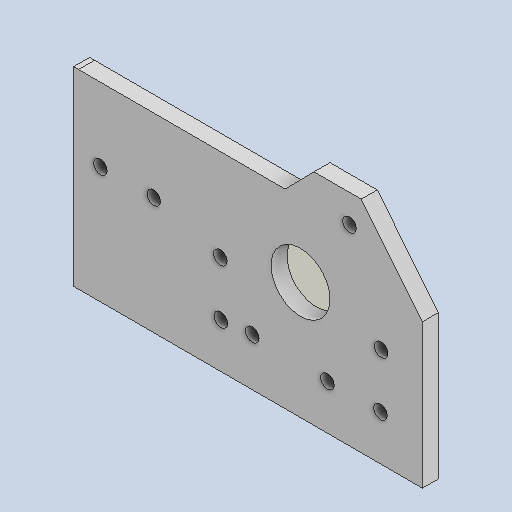
# Autodesk Inventor part: X axis motor mount
Saved by Autodesk Inventor 2023.2 (Build 272271000, 271)
## iProperties
Created: 2023-04-13
Part Number: X axis motor mount
Material: Generic
Document SubType Name: Modeling
Designer: dmargari
Density: 1 g/cm^3
Appearance: Default
Author: dmargari
## iProperties of the stored document X axis motor mount_3DPrint.ipt
Created: 2023-04-13
Part Number: X axis motor mount_3DPrint
Material: Generic
Document SubType Name: Modeling
Designer: dmargari
Density: 1 g/cm^3
Appearance: Default
Author: dmargari
Autodesk Inventor part; units mm, degrees
ref_plane "YZ Plane" through (0, 0, 0) normal (1, 0, 0) x (0, 1, 0)
ref_plane "XZ Plane" through (0, 0, 0) normal (0, 1, 0) x (-1, 0, 0)
ref_plane "XY Plane" through (0, 0, 0) normal (0, 0, 1) x (1, 0, 0)
ref_plane "Work Plane1" through (-0.0001, 0, -396.2798) normal (0.0000002, 0, 1) x (1, 0.0000006, -0.0000002)
sketch "Sketch1" plane through (-0.0001, 0, -396.2798) normal (0.0000002, 0, 1) x (1, 0.0000006, -0.0000002)
  circle A0 centre (29.9617, 10.0469) radius 2.1 projected
  circle A1 centre (29.9617, -9.9531) radius 2.1 projected
  circle A2 centre (-30.0383, -9.9531) radius 2.1 projected
  circle A3 centre (-30.0383, 10.0469) radius 2.1 projected
  circle A4 centre (-10.0383, -9.9531) radius 2.1 projected
  circle A5 centre (9.9617, -9.9531) radius 2.1 projected
  line L0 (39.9617, 19.5469) -> (39.9617, 14.8783) projected
  line L1 (39.9617, -14.7846) -> (39.9617, -19.4531) projected
  line L2 (39.4617, -19.9531) -> (34.7932, -19.9531) projected
  line L3 (20.4617, 20.0469) -> (25.0617, 20.0469) projected
  line L4 (-34.8697, -19.9531) -> (-39.5383, -19.9531) projected
  line L5 (-40.0383, 14.8783) -> (-40.0383, 19.5469) projected
  line L6 (-39.5383, 20.0469) -> (-34.9383, 20.0469) projected
  line L7 (-40.0383, -19.4531) -> (-40.0383, -14.7846) projected
  line L8 (39.9617, 20.0469) -> (39.9617, -19.9532) construction
  line L9 (39.9617, -19.9532) -> (-40.0383, -19.9531) construction
  line L10 (-40.0383, -19.9531) -> (-40.0383, 20.0469) construction
  line L11 (-20.0383, 19.5469) -> (-20.0383, 14.8783) projected
  line L12 (19.9617, 0.0469) -> (19.9617, 5.2154) projected
  line L13 (-20.0383, 0.0469) -> (-14.9383, 0.0469) projected
  line L14 (39.9617, 20.0469) -> (19.9617, 20.0469) construction
  line L15 (19.9617, 20.0469) -> (19.9617, 0.0469) construction
  line L16 (-20.0383, 0.0469) -> (19.9617, 0.0469) construction
  line L17 (-40.0383, 20.0469) -> (-20.0383, 20.0469) construction
  line L18 (-20.0383, 20.0469) -> (-20.0383, 0.0469) construction
  line L19 (45.6493, 27.0762) -> (45.6493, -26.9238)
  line L20 (-64.252, 0) -> (79.446, 0) construction
  line L21 (18.0586, 45.1257) -> (28.1307, -1.0304) construction
  line L22 (28.1307, -1.0304) -> (-18.0254, -11.1025) construction
  circle A6 centre (28.1307, -1.0304) radius 2.55
  circle A7 centre (-18.0452, -9.0596) radius 2.55
  circle A8 centre (18.0586, 45.1257) radius 2.55
  circle A9 centre (-18.0452, -9.0596) radius 3.5 construction
  circle A10 centre (18.0586, 45.1257) radius 3.5 construction
  circle A11 centre (28.1307, -1.0304) radius 3.5 construction
  line L23 (48.593, 17.0469) -> (-85.0986, 17.0469) construction
  line L24 (-0.0383, 40.3857) -> (-0.0383, -33.3677) construction
  circle A12 centre (-0.0383, 17.0469) radius 11.05
  line L25 (45.6493, 27.0762) -> (22.7125, 55.4148)
  line L26 (22.7125, 55.4148) -> (5.0035, 55.4148)
  line L27 (5.0035, 55.4148) -> (-5.8027, 44.4325)
  line L28 (-64.3507, 44.498) -> (-5.8027, 44.4325)
  line L29 (-64.3507, 44.498) -> (-66.5209, 44.5005)
  line L30 (-55.0383, 44.4876) -> (-55.0383, -55.6033) construction
  line L31 (45.6493, -26.9238) -> (-85.0986, -26.7776)
  line L32 (45.6493, -26.9238) -> (185.0342, -26.9238) construction
  line L33 (40.0498, -55.6502) -> (39.9617, -55.6502)
  line L34 (-83.2302, 44.5192) -> (-66.5209, 44.5005)
  line L35 (-85.0986, -26.7776) -> (-85.0986, 44.5192)
  line L36 (-85.0986, 44.5192) -> (-83.2302, 44.5192)
  point P0 (0, 0)
  point P1 (0, 17)
  point P2 (22.7617, 20.0469)
  point P3 (19.9617, 2.6311)
  point P4 (-40.0383, -17.1189)
  point P5 (-55.0383, -5.5579)
  point P6 (-75.0383, 17.0469)
  point P7 (-55.0383, 17.0469)
  dimension "d2" = 110
  dimension "d3" = 5.1
  dimension "d4" = 5.1
  dimension "d5" = 5.1
  dimension "d7" = 7
  dimension "d8" = 7
  dimension "d9" = 7
  dimension "d10" = 3
  dimension "d11" = 20
  dimension "d12" = 22.1
  dimension "d30" = 15
  dimension "d33" = 54
  dimension "d36" = 20
  dimension "d37" = 15
  constraints: 52 end point, 13 coincident, 13 point on line, 7 centre point, 7 perpendicular, 4 horizontal, 4 midpoint, 2 vertical, 1 collinear
  measures "d2" horizontal distance of L28.start L19.start
  measures "d3" diameter of A6
  measures "d4" diameter of A7
  measures "d5" diameter of A8
  measures "d7" diameter of A9
  measures "d8" diameter of A10
  measures "d9" diameter of A11
  measures "d10" distance from line of point (22.762, 20.047) L23
  measures "d11" distance from line of point (19.962, 2.631) L24
  measures "d12" diameter of A12
  measures "d30" distance from line of point (-40.038, -17.119) L30
  measures "d33" distance of L19.start L19.end
  measures "d36" distance of point (-55.038, 17.047) point (-75.038, 17.047)
  measures "d37" distance from line of L10 point (-55.038, 17.047)
extrude "Extrusion1" add sketch "Sketch1" along normal blind 6 contours A0 | A1 | A2 | A3 | A4 | A5 | L19 L31 L35 L36 L34 L29 L28 L27 L26 L25 | A6 | A7 | A8
sketch "Sketch2" plane through (-0.0001, 0, -396.2798) normal (-0.0000002, 0, -1) x (-1, -0.0000006, 0.0000002)
  point P0 (0, 0)
  point P1 (-29.9617, -9.9531)
  point P2 (-10.0691, -10.0439)
  point P3 (9.9252, -10.1028)
  point P4 (18.1169, -8.9461)
  point P5 (29.8554, -9.9987)
  point P6 (30.0649, 10.1011)
  point P7 (-30.1907, 10.308)
  point P8 (-18.3441, 44.9518)
  point P9 (55.0383, 17.0469)
  point P10 (75.0383, 17.0469)
hole "Hole1" at (29.9617, -9.9531, -396.2798) at (10.0691, -10.0439, -396.2798) at (-18.1169, -8.9461, -396.2798) at (-29.8554, -9.9987, -396.2798) at (-30.065, 10.1011, -396.2798) at (30.1907, 10.308, -396.2798) at (18.344, 44.9518, -396.2798) at (-75.0383, 17.0468, -396.2798) at (-55.0383, 17.0468, -396.2798) direction (0.0000002, 0, 1) diameter 5.1 end through all
body "Solid1"
